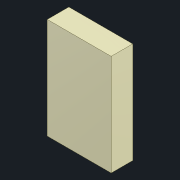
# Autodesk Inventor part: bisco
Saved by Autodesk Inventor 2022 (Build 260153000, 153)
## iProperties
Created: 2021-08-02
Part Number: bisco
Material: bisco
Document SubType Name: Modeling
Designer: yuto6
Density: 0.251397 g/cm^3
Appearance: 滑らか - 灰色
Mass: 85.2698 g
Surface Area: 362.68 cm^2
Volume: 339.184 cm^3
Author: yuto6
Autodesk Inventor part; units mm, degrees
ref_plane "YZ Plane" through (0, 0, 0) normal (1, 0, 0) x (0, 1, 0)
ref_plane "XZ Plane" through (0, 0, 0) normal (0, 1, 0) x (-1, 0, 0)
ref_plane "XY Plane" through (0, 0, 0) normal (0, 0, 1) x (1, 0, 0)
sketch "スケッチ1" plane through (0, 0, 0) normal (0, 0, 1) x (1, 0, 0)
  line L0 (43, 68) -> (-43, 68)
  line L1 (-43, 68) -> (-43, -68)
  line L2 (-43, -68) -> (43, -68)
  line L3 (43, -68) -> (43, 68)
  line L4 (43, 68) -> (-43, -68) construction
  line L5 (-43, 68) -> (43, -68) construction
  point P0 (0, 0)
  dimension "d0" = 136
  dimension "d1" = 86
  constraints: 12 end point, 2 midpoint, 2 parallel, 1 horizontal, 1 perpendicular
  measures "d0" distance of L0.end L1.end
  measures "d1" distance of L0.start L0.end
extrude "押し出し1" add sketch "スケッチ1" along normal blind 29
